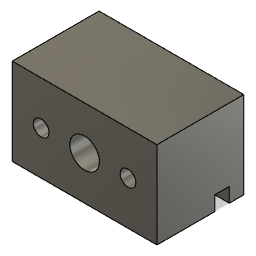
MarkerMount v1 (Autodesk Fusion 360 design; units mm, degrees)
Autodesk Fusion 360 part; units mm, degrees
note: some values were not read from the file. Set by a fixed rule: which sketch regions a step uses.
sketch "Sketch1" plane through (0, 0, 0) normal (0, 0, 1) x (1, 0, 0)
  line L0 (0, 0) -> (50, 0)
  line L1 (50, 0) -> (50, 30)
  line L2 (50, 30) -> (0, 30)
  line L3 (0, 30) -> (0, 0)
  dimension "d1" = 50
  dimension "d2" = 30
  constraint horizontal L0
  constraint vertical L1
  constraint horizontal L2
  constraint vertical L3
  constraint coincident L0.start L3.end
  measures "d1" distance of L0.start L0.end
  measures "d2" distance of L0.start L2.end
extrude "Extrude1" add sketch "Sketch1" along normal blind 30
sketch "Sketch2" plane through (0, 0, 30) normal (0, 0, 1) x (1, 0, 0)
  line L0 (0, 30) -> (0, 0)
  line L1 (0, 0) -> (50, 0)
  line L2 (50, 0) -> (50, 30)
  line L3 (50, 30) -> (0, 30)
  line L4 (0, 30) -> (0, 15)
  line L5 (0, 15) -> (10, 15)
  line L6 (0, 15) -> (25, 15)
  line L7 (50, 15) -> (40, 15)
  circle A0 centre (10, 15) radius 2.725
  circle A1 centre (40, 15) radius 2.725
  circle A2 centre (25, 15) radius 5.125
  dimension "d5" = 10
  dimension "d6" = 25
  dimension "d7" = 10
  dimension "d8" = 5.45
  dimension "d9" = 5.45
  dimension "d10" = 10.25
  constraint coincident L0.start L3.end
  constraint midpoint L0 L4.end
  constraint perpendicular L4 L5
  constraint perpendicular L4 L6
  constraint midpoint L2 L7.start
  constraint perpendicular L2 L7
  constraint coincident L5.end A0.centre
  constraint coincident L7.end A1.centre
  constraint coincident L6.end A2.centre
  measures "d5" distance of L4.end L5.end
  measures "d6" distance of L4.end L6.end
  measures "d7" distance of L7.start L7.end
  measures "d8" diameter of A0
  measures "d9" diameter of A1
  measures "d10" diameter of A2
extrude "Extrude2" cut sketch "Sketch2" against normal blind 30 contours L5 L6 A0 | L5 L6 A0 | A1 | A2
sketch "Sketch3" plane through (0, 0, 0) normal (0, -1, 0) x (1, 0, 0)
  line L0 (0, 0) -> (50, 0)
  line L1 (50, 0) -> (50, 30)
  line L2 (50, 30) -> (0, 30)
  line L3 (0, 30) -> (0, 0)
  line L4 (50, 0) -> (50, 5)
  line L5 (50, 5) -> (25, 5)
  line L6 (25, 5) -> (25, 10)
  line L7 (25, 10) -> (50, 10)
  line L8 (50, 10) -> (50, 5)
  dimension "d13" = 5
  dimension "d14" = 25
  dimension "d15" = 5
  constraint coincident L0.end L1.start
  constraint perpendicular L0 L4
  constraint horizontal L5
  constraint vertical L6
  constraint horizontal L7
  constraint vertical L8
  measures "d13" distance of L0.end L4.end
  measures "d14" distance of L4.end L5.end
  measures "d15" distance of L4.end L7.end
extrude "Extrude3" cut sketch "Sketch3" against normal blind 5 contours L1 L5 L6 L7 L8
